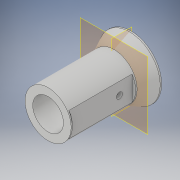
# Autodesk Inventor part: uvlight holder
Saved by Autodesk Inventor 2019 (Build 230136000, 136)
## iProperties
Created: 2019-10-19
Part Number: uvlight holder
Material: Generic
Document SubType Name: Modeling
Designer: Connor Duggan
Density: 1 g/cm^3
Appearance: Default
Author: Connor Duggan
Autodesk Inventor part; units mm, degrees
ref_plane "YZ Plane" through (0, 0, 0) normal (1, 0, 0) x (0, 1, 0)
ref_plane "XZ Plane" through (0, 0, 0) normal (0, 1, 0) x (-1, 0, 0)
ref_plane "XY Plane" through (0, 0, 0) normal (0, 0, 1) x (1, 0, 0)
sketch "Sketch1" plane through (0, 0, 0) normal (0, 0, 1) x (1, 0, 0)
  circle A0 centre (0, 0) radius 23.495
  circle A1 centre (0, 0) radius 25.4
  dimension "d4" = 46.99
  dimension "d5" = 50.8
  constraints: 2 centre point, 2 coincident
  measures "d4" diameter of A0
  measures "d5" diameter of A1
extrude "Extrusion1" add sketch "Sketch1" along normal blind 1.27
ref_plane "Work Plane1" through (0, 0, 13.97) normal (0, 0, 1) x (1, 0, 0)
sketch "Sketch2" plane through (0, 0, 13.97) normal (0, 0, 1) x (1, 0, 0)
  circle A0 centre (0, 0) radius 19.05
  circle A1 centre (0, 0) radius 12.7
  dimension "d9" = 38.1
  dimension "d10" = 25.4
  constraints: 2 centre point, 2 coincident
  measures "d9" diameter of A0
  measures "d10" diameter of A1
sketch "Sketch3" plane through (0, 0, 13.97) normal (0, 0, 1) x (1, 0, 0)
  circle A0 centre (0, 0) radius 10.795 projected
  line L0 (0, 10.795) -> (0, 7.0011) construction
  constraints: 2 end point, 1 vertical, 1 vertical alignment, 1 other
ref_plane "Work Plane2" through (0, 10.795, 13.97) normal (1, 0, 0) x (0, -1, 0)
ref_plane "Work Plane3" through (0, 0, 15.24) normal (0, 0, 1) x (1, 0, 0)
sketch "Sketch5" plane through (0, 0, 15.24) normal (0, 0, 1) x (1, 0, 0)
  circle A0 centre (0, 0) radius 12.7
  circle A1 centre (0, 0) radius 19.05
  dimension "d20" = 38.1
  dimension "d21" = 25.4
  constraints: 2 centre point, 2 coincident
  measures "d20" diameter of A1
  measures "d21" diameter of A0
extrude "Extrusion3" add sketch "Sketch5" along normal blind 50.8
sketch "Sketch6" plane through (0, 10.795, 13.97) normal (1, 0, 0) x (0, -1, 0)
  point P0 (10.795, 13.97)
extrude "Extrusion4" add sketch "Sketch2" along normal blind 1.27
sketch "Sketch7" plane through (0, 10.795, 13.97) normal (1, 0, 0) x (0, -1, 0)
  line L0 (-14.605, 12.7) -> (36.195, 12.7) projected
  line L1 (29.845, 0) -> (-8.255, 0) projected
  line L2 (-14.605, 12.7) -> (-8.255, 0)
  line L3 (-1.905, 0) -> (23.495, 0) projected
  line L4 (-8.255, 0) -> (-1.905, 0)
  line L5 (34.29, 12.7) -> (-12.7, 12.7) projected
  line L6 (-1.905, 0) -> (-12.7, 12.7)
  line L7 (-12.7, 12.7) -> (-14.605, 12.7)
  line L8 (10.795, 0) -> (10.795, 4.3567) construction
  point P0 (10.795, 13.97)
  constraints: 10 end point, 2 collinear, 1 midpoint, 1 vertical
revolve "Revolution2" add sketch "Sketch7" angle 360 about axis through (0, 0, 13.97) along (0, 0, -1)
sketch "Sketch8" plane through (0, 10.795, 13.97) normal (1, 0, 0) x (0, -1, 0)
  point P0 (10.795, 13.97)
sketch "Sketch9" plane through (0, 0, 66.04) normal (0, 0, 1) x (1, 0, 0)
  circle A0 centre (0, 0) radius 19.05 projected
  line L0 (16.0969, 10.1879) -> (16.0969, -10.1879)
  arc A1 (16.0969, -10.1879) -> (16.0969, 10.1879) centre (0, 0) ccw
  constraints: 4 point on circle, 2 end point, 1 centre point, 1 concentric, 1 vertical
extrude "Extrusion5" cut sketch "Sketch9" against normal blind 50.8 contours A0 L0 picked at (16.6372, -2.3328)
sketch "Sketch10" plane through (16.0969, -10.1879, 66.04) normal (1, 0, 0) x (0, 0, -1)
  circle A0 centre (40.3701, 10.1879) radius 2.5
  point P0 (66.04, 10.1879)
  dimension "d24" = 5
  constraints: 1 centre point
  measures "d24" diameter of A0
extrude "Extrusion6" cut sketch "Sketch10" against normal blind 12.7
sketch "Sketch11" plane through (0, 0, 66.04) normal (0, 0, 1) x (1, 0, 0)
  circle A0 centre (0, 0) radius 19.05
  circle A1 centre (0, 0) radius 12.7
  constraints: 2 centre point, 2 coincident
extrude "Extrusion7" add sketch "Sketch11" along normal blind 2.54
chamfer "Chamfer1" distance 1.5875 angle 45 2 edges at (18.2968, 5.3036, 66.04) (18.2968, -5.3036, 66.04)
body "Solid1"
